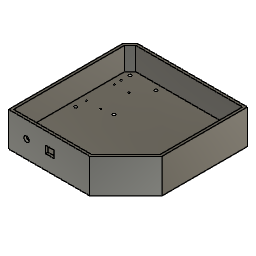
Housing V2-7 (Autodesk Fusion 360 design; units mm, degrees)
Autodesk Fusion 360 part; units mm, degrees
sketch "BoardOutline" plane through (0, 0, 0) normal (0, 0, 1) x (1, 0, 0)
  line L0 (0, 0) -> (101.5, 0)
  line L1 (147, 45.5) -> (147, 152.5)
  line L2 (147, 152.5) -> (7.5, 152.5)
  line L3 (0, 145) -> (0, 0)
  line L4 (7.5, 152.5) -> (0, 145)
  line L5 (147, 45.5) -> (101.5, 0)
  line L6 (7.5, 152.5) -> (7.5, 0) construction
  line L7 (147, 45.5) -> (0, 45.5) construction
  line L8 (101.5, 0) -> (101.5, 152.5) construction
  circle A0 centre (101.5, 45.5) radius 2
  line L9 (0, 145) -> (147, 145) construction
  circle A1 centre (7.5, 145) radius 2
  circle A2 centre (41.5, 145) radius 2
  circle A3 centre (134.5, 145) radius 2
  line L10 (134.5, 152.5) -> (134.5, 33) construction
  circle A4 centre (134.5, 90) radius 2
  circle A5 centre (134.5, 90) radius 2
  circle A6 centre (134.5, 90) radius 2
  circle A7 centre (41.5, 90) radius 2
  circle A8 centre (7.5, 133.5) radius 1.5
  circle A9 centre (7.5, 124.5) radius 1
  circle A10 centre (7.5, 87.5) radius 1
  circle A11 centre (26.5, 124.5) radius 1
  circle A12 centre (26.5, 87.5) radius 1
  circle A13 centre (7.5, 73.5) radius 2
  circle A14 centre (7.5, 7.5) radius 2
  circle A15 centre (131.0677, 63.4488) radius 6 construction
  line L11 (16.5, 0) -> (23.5, 0) construction
  line L12 (23.5, 0) -> (23.5, 13.6837) construction
  line L13 (23.5, 13.6837) -> (16.5, 13.6837) construction
  line L14 (16.5, 13.6837) -> (16.5, 0) construction
  line L15 (96, 0) -> (26, 0) construction
  line L16 (26, 0) -> (26, 82.5) construction
  line L17 (26, 82.5) -> (96, 82.5) construction
  line L18 (96, 82.5) -> (96, 0) construction
  line L19 (55.5, 0) -> (55.5, 10) construction
  line L20 (55.5, 10) -> (45.5, 10) construction
  line L21 (45.5, 10) -> (45.5, 0) construction
  line L22 (45.5, 0) -> (55.5, 0) construction
  line L23 (101.5, 45.5) -> (96, 45.5) construction
  line L24 (55.5, 0) -> (96, 0) construction
  line L25 (51, 130) -> (125, 130) construction
  line L26 (125, 130) -> (125, 105) construction
  line L27 (125, 105) -> (51, 105) construction
  line L28 (51, 105) -> (51, 130) construction
  point P0 (147, 0)
  point P1 (0, 152.5)
  point P2 (7.5, 145)
  point P3 (7.5, 73.5)
  dimension "d1" = 147
  dimension "d2" = 152.5
  dimension "d3" = 7.5
  dimension "d4" = 7.5
  dimension "d5" = 45.5
  dimension "d6" = 45.5
  dimension "d8" = 4
  dimension "d12" = 4
  dimension "d13" = 4
  dimension "d14" = 4
  dimension "d15" = 4
  dimension "d16" = 4
  dimension "d17" = 4
  dimension "d18" = 4
  dimension "d20" = 3
  dimension "d23" = 2
  dimension "d24" = 2
  dimension "d25" = 2
  dimension "d26" = 2
  dimension "d27" = 4
  dimension "d28" = 4
  dimension "d31" = 12
  dimension "d34" = 7
  dimension "d35" = 70
  dimension "d36" = 82.5
  dimension "d39" = 10
  dimension "d40" = 5.5
  dimension "d41" = 93
  dimension "d43" = 55
  dimension "d46" = 34
  constraint horizontal L0
  constraint vertical L1
  constraint horizontal L2
  constraint vertical L3
  constraint coincident L0.start L3.end
  constraint coincident P1 L2
  constraint coincident P1 L3
  constraint coincident P0 L1
  constraint coincident P0 L0
  constraint perpendicular L2 L6
  constraint perpendicular L1 L7
  constraint perpendicular L7 L8
  constraint coincident L8 A0.centre
  constraint coincident L7 A0.centre
  constraint coincident L0 L6.end
  constraint coincident L2 L8.end
  constraint coincident L3 L7.end
  constraint coincident L1 L9.end
  constraint perpendicular L1 L9
  constraint coincident L9 P2
  constraint coincident L6 P2
  constraint coincident L2 L10.start
  constraint coincident L5 L10.end
  constraint perpendicular L2 L10
  constraint coincident P3 A13.centre
  constraint horizontal L11
  constraint vertical L12
  constraint horizontal L13
  constraint vertical L14
  constraint coincident L0 L11.start
  constraint coincident L15 L21.end
  constraint collinear L0 L15
  constraint coincident A0.centre L23.start
  constraint perpendicular L8 L23
  constraint perpendicular L19 L20
  constraint perpendicular L20 L21
  constraint perpendicular L15 L21
  constraint coincident L19 L22.end
  constraint perpendicular L18 L24
  constraint coincident L18 L23.end
  constraint coincident L9 A2.centre
  constraint coincident A3.centre L10
  constraint horizontal L25
  constraint vertical L26
  constraint horizontal L27
  constraint vertical L28
  measures "d1" distance of L0.start P0
  measures "d2" distance of L0.start P1
  measures "d3" distance of P1 L2.end
  measures "d4" distance of P1 L3.start
  measures "d5" distance of P0 L1.start
  measures "d6" distance of P0 L0.end
  measures "d8" diameter of A0
  measures "d12" diameter of A1
  measures "d13" diameter of A2
  measures "d14" diameter of A3
  measures "d15" diameter of A4
  measures "d16" diameter of A5
  measures "d17" diameter of A6
  measures "d18" diameter of A7
  measures "d20" diameter of A8
  measures "d23" diameter of A9
  measures "d24" diameter of A10
  measures "d25" diameter of A11
  measures "d26" diameter of A12
  measures "d27" diameter of A13
  measures "d28" diameter of A14
  measures "d31" diameter of A15
  measures "d34" distance of L11.start L11.end
  measures "d35" distance of L15.start L15.end
  measures "d36" distance of L15.start L17.end
  measures "d39" distance of L19.end L20.end
  measures "d40" distance of A0.centre L23.end
  measures "d41" distance of A2.centre A3.centre
  measures "d43" distance of A3.centre A4.centre
  measures "d46" distance of A2.centre P2
sketch "CasingOutline" plane through (0, 0, 0) normal (0, 0, 1) x (1, 0, 0)
  line L0 (-0.25, -0.25) -> (101.75, -0.25)
  line L1 (147.25, 45.25) -> (147.25, 152.75)
  line L2 (147.25, 152.75) -> (7.25, 152.75)
  line L3 (-0.25, 145.25) -> (-0.25, -0.25)
  line L4 (-3.5, -3.5) -> (103, -3.5)
  line L5 (150.5, 44) -> (150.5, 156)
  line L6 (150.5, 156) -> (5.5, 156)
  line L7 (-3.5, 147) -> (-3.5, -3.5)
  line L8 (147, 152.5) -> (7.5, 152.5)
  line L9 (147.25, 45.25) -> (101.75, -0.25)
  line L10 (-0.25, 145.25) -> (7.25, 152.75)
  line L11 (5.5, 156) -> (-3.5, 147)
  line L12 (150.5, 44) -> (103, -3.5)
  point P0 (147.25, -0.25)
  point P1 (-0.25, 152.75)
  point P2 (150.5, -3.5)
  point P3 (-3.5, 156)
  dimension "d50" = 147.5
  dimension "d51" = 153
  dimension "d52" = 3.25
  dimension "d53" = 3.25
  dimension "d55" = 3.25
  dimension "d56" = 3.25
  dimension "d57" = 45.5
  dimension "d58" = 45.5
  dimension "d59" = 7.5
  dimension "d60" = 7.5
  dimension "d61" = 9
  dimension "d62" = 9
  dimension "d63" = 47.5
  dimension "d64" = 47.5
  constraint horizontal L0
  constraint vertical L1
  constraint horizontal L2
  constraint vertical L3
  constraint horizontal L4
  constraint vertical L5
  constraint horizontal L6
  constraint vertical L7
  constraint coincident P0 L1
  constraint coincident P0 L0
  constraint coincident P1 L3
  constraint coincident P1 L2
  constraint coincident P3 L6
  constraint coincident P3 L7
  constraint coincident P2 L5
  constraint coincident P2 L4
  measures "d50" distance of L0.start P0
  measures "d51" distance of L0.start P1
  measures "d52" distance of L1 L5
  measures "d53" distance of L0 L4
  measures "d55" distance of L2 L6
  measures "d56" distance of L3 L7
  measures "d57" distance of P0 L1.start
  measures "d58" distance of P0 L0.end
  measures "d59" distance of P1 L3.start
  measures "d60" distance of P1 L2.end
  measures "d61" distance of P3 L6.end
  measures "d62" distance of P3 L7.start
  measures "d63" distance of P2 L5.start
  measures "d64" distance of P2 L4.end
extrude "Extrude1" add sketch "CasingOutline" against normal blind 15 contours L0 L1 L2 L3 L9 L10 | L4 L5 L6 L7 L11 L12 makes body 1
extrude "Extrude2" add sketch "CasingOutline" along normal blind 30 bodies 1
hole "Hole1" at (41.5, 90, 0) at (7.5, 73.5, 0) at (41.5, 145, 0) at (7.5, 7.5, 0) at (101.5, 45.5, 0) at (134.5, 90, 0) at (134.5, 145, 0) at (7.5, 145, 0) direction (0, 0, -1) diameter 3.783 depth 10 tip angle 180 bodies 1
thread "Thread1" "ISO Metric profile 4.5 M4.5x0.75 6H"
hole "Hole2" at (7.5, 87.5, 0) at (26.5, 87.5, 0) at (26.5, 124.5, 0) at (7.5, 124.5, 0) direction (0, 0, -1) diameter 2.076 depth 10 tip angle 180 bodies 1
thread "Thread2" "ISO Metric profile 2.5 M2.5x0.45 6H"
hole "Hole3" at (7.5, 133.5, 0) direction (0, 0, -1) diameter 2.529 depth 10 tip angle 180 bodies 1
thread "Thread3" "ISO Metric profile 3.0 M3x0.5 6H"
sketch "IOHoles" plane through (0, -3.5, 0) normal (0, -1, 0) x (1, 0, 0)
  line L0 (-3.5, 30) -> (-3.5, -15)
  line L1 (-3.5, -15) -> (103, -15)
  line L2 (103, -15) -> (103, 30)
  line L3 (103, 30) -> (-3.5, 30)
  circle A0 centre (20, 8) radius 3.5
  line L4 (20, 30) -> (20, -15) construction
  line L5 (45, 13.5) -> (56, 13.5)
  line L6 (56, 13.5) -> (56, 4)
  line L7 (56, 4) -> (45, 4)
  line L8 (45, 4) -> (45, 13.5)
  dimension "d78" = 7
  dimension "d79" = 9.5
  dimension "d80" = 11
  constraint coincident L1 L4.end
  constraint perpendicular L1 L4
  constraint coincident A0.centre L4
  constraint coincident L3 L4.start
  constraint horizontal L5
  constraint vertical L6
  constraint horizontal L7
  constraint vertical L8
  measures "d78" diameter of A0
  measures "d79" distance of L5.end L6.end
  measures "d80" distance of L5.start L5.end
extrude "Extrude3" cut sketch "IOHoles" against normal up to surface (3.25 mm away) contours A0 | L5 L6 L7 L8 bodies 1
sketch "BoardOutline (2)" plane through (0, 0, 0) normal (0, 0, 1) x (1, 0, 0) in component "Lid"
  line L0 (50, 135) -> (125, 135)
  line L1 (125, 135) -> (125, 105)
  circle A0 centre (134.5, 90) radius 2
  line L2 (147, 45.5) -> (101.5, 0)
  line L3 (147, 152.5) -> (7.5, 152.5)
  line L4 (0, 0) -> (101.5, 0)
  line L5 (147, 45.5) -> (0, 45.5) construction
  line L6 (0, 145) -> (147, 145) construction
  line L7 (101.5, 45.5) -> (96, 45.5) construction
  circle A1 centre (134.5, 90) radius 2
  circle A2 centre (134.5, 90) radius 2
  line L8 (134.5, 152.5) -> (134.5, 33) construction
  circle A3 centre (134.5, 145) radius 2
  circle A4 centre (120, 70) radius 10
  circle A5 centre (101.5, 45.5) radius 2
  line L9 (26, 82.5) -> (96, 82.5) construction
  line L10 (45.5, 0) -> (55.5, 0) construction
  circle A6 centre (7.5, 145) radius 2
  line L11 (16.5, 13.6837) -> (16.5, 0) construction
  line L12 (55.5, 0) -> (55.5, 10) construction
  line L13 (96, 0) -> (26, 0) construction
  line L14 (50, 105) -> (50, 135)
  line L15 (23.5, 0) -> (23.5, 13.6837) construction
  circle A7 centre (41.5, 145) radius 2
  circle A8 centre (7.5, 87.5) radius 1
  line L16 (16.5, 0) -> (23.5, 0) construction
  circle A9 centre (26.5, 124.5) radius 1
  circle A10 centre (7.5, 124.5) radius 1
  line L17 (55.5, 0) -> (96, 0) construction
  circle A11 centre (7.5, 73.5) radius 2
  line L18 (55.5, 10) -> (45.5, 10) construction
  circle A12 centre (7.5, 133.5) radius 1.5
  line L19 (7.5, 152.5) -> (0, 145)
  circle A13 centre (7.5, 7.5) radius 2
  circle A14 centre (41.5, 90) radius 2
  line L20 (45.5, 10) -> (45.5, 0) construction
  circle A15 centre (26.5, 87.5) radius 1
  line L21 (23.5, 13.6837) -> (16.5, 13.6837) construction
  line L22 (0, 145) -> (0, 0)
  line L23 (96, 82.5) -> (96, 0) construction
  line L24 (26, 0) -> (26, 82.5) construction
  line L25 (7.5, 152.5) -> (7.5, 0) construction
  line L26 (101.5, 0) -> (101.5, 152.5) construction
  line L27 (125, 105) -> (50, 105)
  line L28 (147, 45.5) -> (147, 152.5)
  point P0 (7.5, 73.5)
  point P1 (0, 152.5)
  point P2 (147, 0)
  point P3 (7.5, 145)
  dimension "d84" = 147
  dimension "d85" = 152.5
  dimension "d86" = 7.5
  dimension "d87" = 7.5
  dimension "d88" = 45.5
  dimension "d89" = 45.5
  dimension "d90" = 4
  dimension "d91" = 4
  dimension "d92" = 4
  dimension "d93" = 4
  dimension "d94" = 4
  dimension "d95" = 4
  dimension "d96" = 4
  dimension "d97" = 4
  dimension "d98" = 3
  dimension "d99" = 2
  dimension "d100" = 2
  dimension "d101" = 2
  dimension "d102" = 2
  dimension "d103" = 4
  dimension "d104" = 4
  dimension "d105" = 20
  dimension "d106" = 7
  dimension "d107" = 70
  dimension "d108" = 82.5
  dimension "d109" = 10
  dimension "d110" = 5.5
  dimension "d111" = 93
  dimension "d112" = 55
  dimension "d113" = 34
  constraint horizontal L4
  constraint vertical L28
  constraint horizontal L3
  constraint vertical L22
  constraint coincident L4.start L22.end
  constraint coincident P1 L3
  constraint coincident P1 L22
  constraint coincident P2 L28
  constraint coincident P2 L4
  constraint perpendicular L3 L25
  constraint perpendicular L5 L28
  constraint perpendicular L5 L26
  constraint coincident L7.start L26
  constraint coincident L7.start L5
  constraint coincident L25.end L4
  constraint coincident L26.end L3
  constraint coincident L5.end L22
  constraint coincident L6.end L28
  constraint perpendicular L6 L28
  constraint coincident P3 L6
  constraint coincident P3 L25
  constraint coincident L8.start L3
  constraint coincident L8.end L2
  constraint perpendicular L3 L8
  constraint coincident P0 A11.centre
  constraint horizontal L16
  constraint vertical L15
  constraint horizontal L21
  constraint vertical L11
  constraint coincident L11.end L4
  constraint coincident L10.start L13
  constraint collinear L4 L13
  constraint coincident L7.start A5.centre
  constraint perpendicular L7 L26
  constraint perpendicular L12 L18
  constraint perpendicular L18 L20
  constraint perpendicular L13 L20
  constraint coincident L10.end L12
  constraint perpendicular L17 L23
  constraint coincident L7.end L23
  constraint coincident A7.centre L6
  constraint coincident A3.centre L8
  constraint horizontal L0
  constraint vertical L1
  constraint horizontal L27
  constraint vertical L14
  measures "d84" distance of P2 L4.start
  measures "d85" distance of P1 L4.start
  measures "d86" distance of L3.end P1
  measures "d87" distance of L6.start P1
  measures "d88" distance of L2.start P2
  measures "d89" distance of L2.end P2
  measures "d90" diameter of A5
  measures "d91" diameter of A6
  measures "d92" diameter of A7
  measures "d93" diameter of A3
  measures "d94" diameter of A2
  measures "d95" diameter of A1
  measures "d96" diameter of A0
  measures "d97" diameter of A14
  measures "d98" diameter of A12
  measures "d99" diameter of A10
  measures "d100" diameter of A8
  measures "d101" diameter of A9
  measures "d102" diameter of A15
  measures "d103" diameter of A11
  measures "d104" diameter of A13
  measures "d105" diameter of A4
  measures "d106" distance of L15.start L11.end
  measures "d107" distance of L13.end L13.start
  measures "d108" distance of L9.end L13.start
  measures "d109" distance of L18.end L12.end
  measures "d110" distance of L7.end L7.start
  measures "d111" distance of A3.centre A7.centre
  measures "d112" distance of A3.centre A0.centre
  measures "d113" distance of A7.centre P3
sketch "CasingOutline (2)" plane through (0, 0, 0) normal (0, 0, 1) x (1, 0, 0) in component "Lid"
  line L0 (147.25, 45.25) -> (101.75, -0.25)
  line L1 (147.25, 152.75) -> (7.25, 152.75)
  line L2 (-0.25, -0.25) -> (101.75, -0.25)
  line L3 (150.5, 44) -> (103, -3.5)
  line L4 (-0.25, 145.25) -> (7.25, 152.75)
  line L5 (5.5, 156) -> (-3.5, 147)
  line L6 (-3.5, 147) -> (-3.5, -3.5)
  line L7 (150.5, 156) -> (5.5, 156)
  line L8 (147, 152.5) -> (7.5, 152.5)
  line L9 (-0.25, 145.25) -> (-0.25, -0.25)
  line L10 (147.25, 45.25) -> (147.25, 152.75)
  line L11 (-3.5, -3.5) -> (103, -3.5)
  line L12 (150.5, 44) -> (150.5, 156)
  point P0 (-3.5, 156)
  point P1 (150.5, -3.5)
  point P2 (147.25, -0.25)
  point P3 (-0.25, 152.75)
  dimension "d114" = 147.5
  dimension "d115" = 153
  dimension "d116" = 3.25
  dimension "d117" = 3.25
  dimension "d118" = 3.25
  dimension "d119" = 3.25
  dimension "d120" = 45.5
  dimension "d121" = 45.5
  dimension "d122" = 7.5
  dimension "d123" = 7.5
  dimension "d124" = 9
  dimension "d125" = 9
  dimension "d126" = 47.5
  dimension "d127" = 47.5
  constraint horizontal L2
  constraint vertical L10
  constraint horizontal L1
  constraint vertical L9
  constraint horizontal L11
  constraint vertical L12
  constraint horizontal L7
  constraint vertical L6
  constraint coincident P2 L10
  constraint coincident P2 L2
  constraint coincident P3 L9
  constraint coincident P3 L1
  constraint coincident P0 L7
  constraint coincident P0 L6
  constraint coincident P1 L12
  constraint coincident P1 L11
  measures "d114" distance of P2 L2.start
  measures "d115" distance of P3 L2.start
  measures "d116" distance of L10 L12
  measures "d117" distance of L2 L11
  measures "d118" distance of L1 L7
  measures "d119" distance of L6 L9
  measures "d120" distance of P2 L0.start
  measures "d121" distance of P2 L0.end
  measures "d122" distance of P3 L4.start
  measures "d123" distance of L1.end P3
  measures "d124" distance of P0 L5.start
  measures "d125" distance of P0 L5.end
  measures "d126" distance of P1 L3.start
  measures "d127" distance of P1 L3.end
extrude "Extrude1'" add sketch "CasingOutline" along normal blind 5 separate body contours L0 L1 L2 L3 L9 L10 | L4 L5 L6 L7 L11 L12 makes body 2 in component "Lid"
extrude "Extrude2'" add sketch "CasingOutline (2)" against normal blind 3 contours L0 L1 L2 L4 L9 L10 bodies 2 in component "Lid"
move_face "OffsetFaces1" offset -1 5 faces at (-0.25, 96.75, -1) (33.75, -0.25, -2) (147.25, 81.0833, -1) (132.0833, 30.0833, -1) (100.5833, 152.75, -1) on bodies 2 in component "Lid"
move_body "Move1" bodies 2 to x (1, 0, 0) y (0, 1, 0) z (0, 0, 1) at (0, 0, -5) in component "Lid"
extrude "Extrude3'" cut sketch "BoardOutline (2)" against normal up to surface (8 mm away) contours L0 L1 L14 L27 | A0 A1 A2 | A3 | A4 | A5 | A6 | A7 | A11 | A12 | A13 | A14 bodies 2 in component "Lid"
move_body "Move2" bodies 2 to x (1, 0, 0) y (0, 1, 0) z (0, 0, 1) at (0, 0, 35) in component "Lid"
component "Lid" placed x (1, 0, 0) y (0, 1, 0) z (0, 0, 1) at (0, 0, 0)
equation "d4 = d3"
equation "d6 = d5"
equation "d58 = d57"
equation "d60 = d59"
equation "d62 = d61"
equation "d64 = d63"
equation "d87 = d3"
equation "d89 = d5"
equation "d121 = d57"
equation "d123 = d59"
equation "d125 = d61"
equation "d127 = d63"
